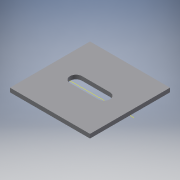
# Autodesk Inventor part: top
Saved by Autodesk Inventor 2018 (Build 220112000, 112)
## iProperties
Created: 2018-01-08
Part Number: top
Material: Generic
Document SubType Name: Modeling
Designer: erwin
Density: 1 g/cm^3
Appearance: Default
Author: erwin
Autodesk Inventor part; units mm, degrees
ref_plane "YZ Plane" through (0, 0, 0) normal (1, 0, 0) x (0, 1, 0)
ref_plane "XZ Plane" through (0, 0, 0) normal (0, 1, 0) x (-1, 0, 0)
ref_plane "XY Plane" through (0, 0, 0) normal (0, 0, 1) x (1, 0, 0)
ref_plane "Work Plane1" through (0, 0, 0) normal (0, 0, 1) x (1, 0, 0)
sketch "Sketch1" plane through (0, 0, 0) normal (0, 0, 1) x (1, 0, 0)
  line L0 (-8, 18) -> (8, 18) projected
  line L1 (8, 18) -> (8, 2) projected
  line L2 (8, 2) -> (-8, 2) projected
  line L3 (-8, 2) -> (-8, 18) projected
  line L4 (10, 20) -> (-10, 20) projected
  line L5 (-10, 0) -> (-10, 20) projected
  line L6 (10, 0) -> (-10, 0) projected
  line L7 (10, 20) -> (10, 0) projected
  point P0 (0, 0)
extrude "Extrusion1" add sketch "Sketch1" along normal blind 1 contours L0 L1 L2 L3 | L7 L6 L5 L4
sketch "Sketch2" plane through (0, 0, 1) normal (0, 0, 1) x (1, 0, 0)
  line L0 (5, 10) -> (-5, 10) construction
  line L1 (3.5, 11.5) -> (-3.5, 11.5)
  line L2 (-3.5, 8.5) -> (3.5, 8.5)
  arc A0 (3.5, 8.5) -> (3.5, 11.5) centre (3.5, 10) ccw
  arc A1 (-3.5, 11.5) -> (-3.5, 8.5) centre (-3.5, 10) ccw
  line L3 (10, 20) -> (-10, 20) projected
  line L4 (-10, 20) -> (-10, 0) projected
  line L5 (10, 0) -> (10, 20) projected
  line L6 (-10, 0) -> (10, 0) projected
  point P0 (0, 0)
  point P1 (0, 10)
  dimension "d2" = 10
  dimension "d3" = 3
  dimension "d4" = 8.5
  dimension "d5" = 5
  dimension "d6" = 5
  dimension "d7" = 8.5
  constraints: 8 end point, 6 point on circle, 4 tangent, 2 centre point, 2 point on line, 1 horizontal, 1 midpoint, 1 parallel
  measures "d2" distance of L0.start L0.end
  measures "d3" diameter of A1
  measures "d4" distance between parallel lines of L3 L1
  measures "d5" distance from line of L4 L0.end
  measures "d6" distance from line of L5 L0.start
  measures "d7" distance between parallel lines of L6 L2
extrude "Extrusion2" cut sketch "Sketch2" against normal through all contours A0 L2 A1 L1
equation "\"d4\" = d7"
equation "\"d5\" = d6"
body "Solid1"
